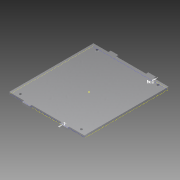
# Autodesk Inventor part: BottomPlate
Saved by Autodesk Inventor 2015 SP1 (Build 190203100, 203)
## iProperties
Created: 2015-01-22
Part Number: BottomPlate
Material: Acrylic, Clear
Document SubType Name: Modeling
Designer: Patrick
Density: 1.19 g/cm^3
Appearance: Transparent - Clear
Author: Patrick
Autodesk Inventor part; units mm, degrees
ref_plane "YZ Plane" through (0, 0, 0) normal (1, 0, 0) x (0, 1, 0)
ref_plane "XZ Plane" through (0, 0, 0) normal (0, 1, 0) x (-1, 0, 0)
ref_plane "XY Plane" through (0, 0, 0) normal (0, 0, 1) x (1, 0, 0)
sketch "Sketch1" plane through (0, 0, 0) normal (0, 0, 1) x (1, 0, 0)
  line L0 (-50, 56) -> (50, 56)
  line L1 (50, 56) -> (50, -56)
  line L2 (50, -56) -> (-50, -56)
  line L3 (-50, -56) -> (-50, 56)
  line L4 (-50, 56) -> (50, -56) construction
  line L5 (50, 56) -> (-50, -56) construction
  point P0 (0, 0)
  point P1 (0, 0)
  point P2 (0, 0)
  dimension "d0" = 100
  dimension "d1" = 112
  constraints: 12 end point, 3 midpoint, 2 parallel, 1 coincident, 1 horizontal, 1 perpendicular
  measures "d0" distance of L1.end L2.end
  measures "d1" distance of L0.end L1.end
extrude "Extrusion1" add sketch "Sketch1" along normal blind 3
sketch "Sketch2" plane through (0, 0, 3) normal (0, 0, 1) x (1, 0, 0)
  line L0 (-50, -56) -> (50, -56) projected
  line L1 (-30.065, -59) -> (-19.935, -59)
  line L2 (-19.935, -59) -> (-19.935, -56)
  line L3 (-19.935, -56) -> (-30.065, -56)
  line L4 (-30.065, -56) -> (-30.065, -59)
  line L5 (-30.065, -59) -> (-19.935, -56) construction
  line L6 (-19.935, -59) -> (-30.065, -56) construction
  line L7 (19.935, -59) -> (30.065, -59)
  line L8 (30.065, -59) -> (30.065, -56)
  line L9 (30.065, -56) -> (19.935, -56)
  line L10 (19.935, -56) -> (19.935, -59)
  line L11 (19.935, -59) -> (30.065, -56) construction
  line L12 (30.065, -59) -> (19.935, -56) construction
  point P0 (0, 0)
  point P1 (-25, -57.5)
  point P2 (25, -57.5)
  dimension "d4" = 3
  dimension "d5" = 25
  dimension "d6" = 25
  dimension "d7" = 10.13
  dimension "d8" = 10.13
  constraints: 24 end point, 4 midpoint, 4 parallel, 2 horizontal, 2 perpendicular, 2 point on line, 1 collinear
  measures "d4" distance of L3.end L1.start
  measures "d5" horizontal distance of point (0, 0) point (-25, -57.5)
  measures "d6" horizontal distance of point (25, -57.5) point (0, 0)
  measures "d7" distance of L1.start L1.end
  measures "d8" distance of L7.start L7.end
extrude "Extrusion2" add sketch "Sketch2" against normal blind 3
mirror "Mirror1" about plane through (0, 0, 0) normal (0, 1, 0) of "Extrusion2"
sketch "Sketch3" plane through (0, 0, 0) normal (0, 0, -1) x (-1, 0, 0)
  line L0 (-50, -56) -> (-50, 56) construction
  line L1 (-50, 55) -> (50, 55) construction
  line L2 (50, 56) -> (50, -56) construction
  line L3 (-50, -55) -> (50, -55) construction
  line L4 (-19.935, -56) -> (19.935, -56) construction
  line L5 (-30.065, 56) -> (-50, 56) construction
  point P0 (0, 0)
  dimension "d11" = 1
  dimension "d12" = 1
  constraints: 4 end point, 4 point on line, 1 horizontal, 1 perpendicular
  measures "d11" distance between parallel lines of L4 L3
  measures "d12" distance between parallel lines of L5 L1
ref_plane "Work Plane1" through (-19.935, -55, 0) normal (0, -1, 0) x (1, 0, 0)
sketch "Sketch4" plane through (0, 0, 3) normal (0, 0, 1) x (1, 0, 0)
  line L0 (-50, 56) -> (-50, -56) projected
  line L1 (-50, -56) -> (-30.065, -56) projected
  line L2 (-30.065, 56) -> (-50, 56) projected
  line L3 (50, -56) -> (50, 56) projected
  point P0 (0, 0)
  point P1 (-40.1, -50.9)
  point P2 (-40.1, 50.9)
  point P3 (40.9, -50.9)
  point P4 (40.9, 50.9)
  dimension "d14" = 9.9
  dimension "d15" = 5.1
  dimension "d16" = 5.1
  dimension "d17" = 9.1
  constraints: 2 horizontal alignment, 2 vertical alignment
  measures "d14" distance from line of point (-40.1, -50.9) L0
  measures "d15" distance from line of L1 point (-40.1, -50.9)
  measures "d16" distance from line of L2 point (-40.1, 50.9)
  measures "d17" distance from line of point (40.9, -50.9) L3
hole "Hole2" at (-40.1, -50.9, 3) at (40.9, -50.9, 3) at (40.9, 50.9, 3) at (-40.1, 50.9, 3) direction (0, 0, -1) diameter 3 end through all
equation "\"d6\" = d5"
equation "\"d8\" = d7"
equation "\"d12\" = d11"
equation "\"d16\" = d15"
equation "\"kerf\" = 0.13"
body "Solid1"
